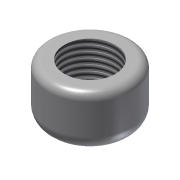
# Autodesk Inventor part: HANDLE CAP
Saved by Autodesk Inventor 2014 (Build 180170000, 170)
## iProperties
Created: 2014-12-22
Part Number: HANDLE CAP
Material: Steel, Mild
Document SubType Name: Modeling
Designer: Ebrahim
Density: 7.86 g/cm^3
Appearance: Steel
Mass: 24.2057 g
Surface Area: 18.4826 cm^2
Volume: 3.0796 cm^3
Author: Ebrahim
Autodesk Inventor part; units mm, degrees
ref_plane "YZ Plane" through (0, 0, 0) normal (1, 0, 0) x (0, 1, 0)
ref_plane "XZ Plane" through (0, 0, 0) normal (0, 1, 0) x (-1, 0, 0)
ref_plane "XY Plane" through (0, 0, 0) normal (0, 0, 1) x (1, 0, 0)
sketch "Sketch1" plane through (0, 0, 0) normal (0, 0, 1) x (1, 0, 0)
  circle A0 centre (0, 0) radius 11
  dimension "d0" = 22
  constraints: 1 centre point, 1 coincident
  measures "d0" diameter of A0
extrude "Extrusion1" add sketch "Sketch1" along normal blind 14
fillet "Fillet1" radius 2 1 edges at (-11, 0, 14)
fillet "Fillet1" radius 4 1 edges at (-11, 0, 0)
hole "Hole1" at (0, 0, 14) direction (0, 0, -1) diameter 13.376 end through all thread size "M15x1.5" class "6H" standard "ISO Metric profile"
body "Solid1"
